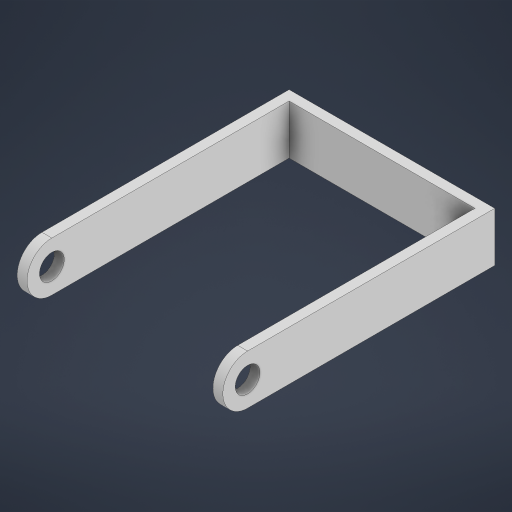
# Autodesk Inventor part: gunholder_clip
Saved by Autodesk Inventor 2024 (Build 280153000, 153)
## iProperties
Created: 2023-06-15
Part Number: gunholder_clip
Material: 일반
Document SubType Name: Modeling
Designer: 6gioc
Density: 1 g/cm^3
Appearance: 기본값
Author: 6gioc
Autodesk Inventor part; units mm, degrees
ref_plane "YZ Plane" through (0, 0, 0) normal (1, 0, 0) x (0, 1, 0)
ref_plane "XZ Plane" through (0, 0, 0) normal (0, 1, 0) x (-1, 0, 0)
ref_plane "XY Plane" through (0, 0, 0) normal (0, 0, 1) x (1, 0, 0)
sketch "스케치1" plane through (0, 0, 0) normal (1, 0, 0) x (0, 1, 0)
  circle A0 centre (0, 0) radius 2.5
  circle A1 centre (0, 0) radius 5
  line L0 (5, 0) -> (-5, 0)
  line L1 (-5, 0) -> (-5, -50)
  line L2 (-5, -50) -> (5, -50)
  line L3 (5, -50) -> (5, 0)
  dimension "d1" = 10
  dimension "d0" = 5
  dimension "d2" = 10
  dimension "d3" = 50
  constraints: 8 end point, 2 coincident, 2 parallel, 1 centre point, 1 horizontal, 1 perpendicular, 3 other
  measures "d0" diameter of A0
  measures "d2" distance of L2.end L1.end
  measures "d3" distance of L1.end L0.end
extrude "돌출1" add sketch "스케치1" along normal blind 2 contours L0 A1 A0 | A0 L0 A1 | L3 L2 L1 A1
sketch "스케치2" plane through (0, 0, 0) normal (-1, 0, 0) x (0, 0, 1)
  line L0 (-50, -5) -> (-50, 5) projected
  line L1 (-50, 5) -> (-48, 5)
  line L2 (-48, 5) -> (-48, -5)
  line L3 (-48, -5) -> (-50, -5)
  line L4 (-50, -5) -> (-50, 5)
  point P0 (0, 0)
  dimension "d6" = 2
  dimension "d7" = 10
  constraints: 8 end point, 2 parallel, 1 horizontal, 1 perpendicular
  measures "d6" distance of L2.end L3.end
  measures "d7" distance of L1.end L2.end
extrude "돌출2" add sketch "스케치2" along normal blind 37.6
sketch "스케치3" plane through (-37.6, 0, 0) normal (-1, 0, 0) x (0, 0, 1)
  line L0 (-50, -5) -> (-50, 5) projected
  line L1 (0, -5) -> (-50, -5) projected
  line L2 (-50, 5) -> (0, 5)
  line L3 (0, 5) -> (0, -5)
  line L4 (0, -5) -> (-50, -5)
  line L5 (-50, -5) -> (-50, 5)
  circle A0 centre (0, 0) radius 5
  circle A1 centre (0, 0) radius 2.5
  dimension "d10" = 50
  dimension "d11" = 10
  dimension "d12" = 5
  constraints: 8 end point, 2 centre point, 2 coincident, 2 parallel, 1 horizontal, 1 perpendicular, 1 tangent
  measures "d10" distance of L1.start L4.end
  measures "d11" distance of L2.end L1.start
  measures "d12" diameter of A1
extrude "돌출3" add sketch "스케치3" along normal blind 2 contours L0 L2 A0 L1 | A0 L3 A1 | L3 A1 A0
